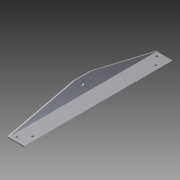
# Autodesk Inventor part: 8 ball top lift point
Saved by Autodesk Inventor 2012 (Build 160160000, 160)
## iProperties
Created: 2013-11-12
Part Number: 8 ball top lift point
Material: Default
Document SubType Name: Modeling
Designer: Bryce
Density: 1 g/cm^3
Author: Bryce
Autodesk Inventor part; units mm, degrees
ref_plane "YZ Plane" through (0, 0, 0) normal (1, 0, 0) x (0, 1, 0)
ref_plane "XZ Plane" through (0, 0, 0) normal (0, 1, 0) x (-1, 0, 0)
ref_plane "XY Plane" through (0, 0, 0) normal (0, 0, 1) x (1, 0, 0)
sketch "Sketch1" plane through (0, 0, 0) normal (0, 0, 1) x (1, 0, 0)
  line L0 (0, 0) -> (25.4, 0)
  line L1 (25.4, 0) -> (25.4, 25.4)
  line L2 (25.4, 25.4) -> (0, 25.4)
  line L3 (0, 25.4) -> (0, 0)
  line L4 (25.4, 25.4) -> (1.5875, 25.4)
  line L5 (1.5875, 25.4) -> (1.5875, 1.5875)
  line L6 (1.5875, 1.5875) -> (25.4, 1.5875)
  line L7 (25.4, 1.5875) -> (25.4, 25.4)
  dimension "d0" = 1.5875
  dimension "d1" = 1.5875
  dimension "d2" = 25.4
  dimension "d3" = 25.4
  constraints: 16 end point, 4 parallel, 2 horizontal, 2 perpendicular
  measures "d0" distance between parallel lines of L0 L6
  measures "d1" distance between parallel lines of L3 L5
  measures "d2" distance of L0.start L0.end
  measures "d3" distance of L2.end L0.start
extrude "Extrusion1" add sketch "Sketch1" along normal blind 225.425 contours L3 L2 L5 L6 L1 L0
sketch "Sketch2" plane through (0, 0, 0) normal (0, -1, 0) x (1, 0, 0)
  line L0 (25.4, 225.425) -> (0, 225.425) projected
  line L1 (0, 0) -> (0, 225.425) projected
  line L2 (25.4, 0) -> (25.4, 225.425) projected
  circle A0 centre (7.9375, 219.075) radius 1.5875
  circle A1 centre (19.05, 206.375) radius 1.5875
  line L3 (0, 112.7125) -> (25.4, 112.7125)
  circle A2 centre (7.9375, 6.35) radius 1.5875
  circle A3 centre (19.05, 19.05) radius 1.5875
  dimension "d6" = 3.175
  dimension "d7" = 6.35
  dimension "d8" = 7.9375
  dimension "d9" = 19.05
  dimension "d10" = 6.35
  constraints: 4 centre point, 2 end point, 2 midpoint, 2 symmetric about line, 1 equal radius, 2 other
  measures "d6" diameter of A0
  measures "d7" distance from line of L0 A0.centre
  measures "d8" distance from line of L1 A0.centre
  measures "d9" distance from line of L0 A1.centre
  measures "d10" distance from line of L2 A1.centre
extrude "Extrusion2" cut sketch "Sketch2" against normal blind 225.425 contours A0 | A1 | A2 | A3
sketch "Sketch3" plane through (0, 0, 0) normal (-1, 0, 0) x (0, 0, 1)
  line L0 (225.425, 0) -> (225.425, 25.4) projected
  line L1 (0, 25.4) -> (225.425, 25.4) projected
  line L2 (0, 25.4) -> (0, 0) projected
  line L3 (0, 0) -> (225.425, 0) projected
  circle A0 centre (112.7125, 15.875) radius 3.175
  line L4 (0, 1.5875) -> (100.0125, 25.4)
  line L5 (125.4125, 25.4) -> (225.425, 1.5875)
  dimension "d13" = 6.35
  dimension "d14" = 15.875
  dimension "d15" = 112.7125
  dimension "d16" = 1.5875
  dimension "d17" = 1.5875
  dimension "d18" = 12.7
  dimension "d19" = 25.4
  constraints: 4 end point, 4 point on line, 1 centre point
  measures "d13" diameter of A0
  measures "d14" distance from line of L3 A0.centre
  measures "d15" distance from line of L2 A0.centre
  measures "d16" distance of L2.end L4.start
  measures "d17" distance of L0.start L5.end
  measures "d18" horizontal distance of A0.centre L4.end
  measures "d19" distance of L4.end L5.start
extrude "Extrusion3" cut sketch "Sketch3" against normal blind 225.425 contours L5 L1 L0 | L2 L1 L4 | A0
equation "\"d0\" = d1"
equation "\"d3\" = d2"
equation "\"d18\" = 0.5 * d19"
body "Solid1"
